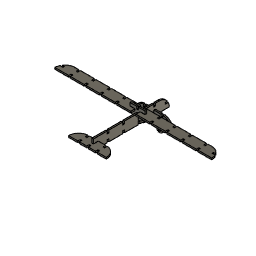
Pressfit Construction Kit v5 (Autodesk Fusion 360 design; units mm, degrees)
Autodesk Fusion 360 part; units mm, degrees
sketch "Sketch1" plane through (0, 0, 0) normal (0, 0, 1) x (1, 0, 0)
  line L0 (75, -10) -> (-75, -10)
  line L1 (-55, 10) -> (75, 10)
  arc A0 (-55, 10) -> (-75, -10) centre (-55, -10) ccw
  line L2 (0, 48.6759) -> (0, -48.6759)
  arc A1 (75, -10) -> (55, 10) centre (55, -10) ccw
  line L3 (-47.4, -10) -> (-44.4, -10)
  line L4 (-44.4, -10) -> (-44.4, -5)
  line L5 (-44.4, -5) -> (-47.4, -5)
  line L6 (-47.4, -5) -> (-47.4, -10)
  line L7 (-13.8, -5) -> (-16.8, -5)
  line L8 (-16.8, -10) -> (-13.8, -10)
  line L9 (-16.8, -5) -> (-16.8, -10)
  line L10 (-13.8, -10) -> (-13.8, -5)
  line L11 (16.8, -5) -> (13.8, -5)
  line L12 (13.8, -10) -> (16.8, -10)
  line L13 (13.8, -5) -> (13.8, -10)
  line L14 (16.8, -10) -> (16.8, -5)
  line L15 (47.4, -5) -> (44.4, -5)
  line L16 (44.4, -10) -> (47.4, -10)
  line L17 (44.4, -5) -> (44.4, -10)
  line L18 (47.4, -10) -> (47.4, -5)
  line L19 (-75, -10) -> (-75, 10) construction
  line L20 (-47.4, -7.5) -> (-75, -7.5) construction
  line L21 (47.4, -7.5) -> (75, -7.5) construction
  line L22 (75, -10) -> (75, 10)
  line L23 (-44.4, -7.5) -> (-16.8, -7.5) construction
  line L24 (-13.8, -7.5) -> (13.8, -7.5) construction
  line L25 (16.8, -7.5) -> (44.4, -7.5) construction
  line L26 (-89.7829, 0) -> (89.7829, 0)
  line L27 (16.8, 5) -> (13.8, 5)
  line L28 (13.8, 10) -> (16.8, 10)
  line L29 (-16.8, 5) -> (-16.8, 10)
  line L30 (-44.4, 10) -> (-44.4, 5)
  line L31 (-13.8, 5) -> (-16.8, 5)
  line L32 (44.4, 5) -> (44.4, 10)
  line L33 (-16.8, 10) -> (-13.8, 10)
  line L34 (16.8, 10) -> (16.8, 5)
  line L35 (13.8, 5) -> (13.8, 10)
  line L36 (-44.4, 5) -> (-47.4, 5)
  line L37 (47.4, 5) -> (44.4, 5)
  line L38 (-47.4, 5) -> (-47.4, 10)
  line L39 (44.4, 10) -> (47.4, 10)
  line L40 (-47.4, 10) -> (-44.4, 10)
  line L41 (-13.8, 10) -> (-13.8, 5)
  line L42 (47.4, 10) -> (47.4, 5)
  line L43 (-67.3205, -1.5) -> (-77.3205, -1.5)
  line L44 (-77.3205, -1.5) -> (-77.3205, 1.5)
  line L45 (-77.3205, 1.5) -> (-67.3205, 1.5)
  line L46 (-67.3205, 1.5) -> (-67.3205, -1.5)
  line L47 (-67.3205, -1.5) -> (-77.3205, 1.5) construction
  line L48 (-77.3205, -1.5) -> (-67.3205, 1.5) construction
  line L49 (75, 1.5) -> (70, 1.5)
  line L50 (70, 1.5) -> (70, -1.5)
  line L51 (70, -1.5) -> (75, -1.5)
  line L52 (75, -1.5) -> (75, 1.5)
  point P0 (44.4, 7.5)
  point P1 (-13.8, 7.5)
  point P2 (13.8, 7.5)
  point P3 (47.4, 7.5)
  point P4 (-16.8, 7.5)
  point P5 (-44.4, 7.5)
  point P6 (-47.4, 7.5)
  point P7 (16.8, 7.5)
  point P8 (55, 10)
  point P9 (-55, 10)
  point P10 (-72.3205, 0)
  dimension "d3" = 150
  dimension "d4" = 20
  dimension "d5" = 20
  dimension "d6" = 10
  dimension "d7" = 110
  dimension "d12" = 3
  dimension "d13" = 5
  dimension "d27" = 3
  dimension "d28" = 10
  dimension "d29" = 5
  dimension "d30" = 3
  constraint horizontal L0
  constraint parallel L0 L1
  constraint perpendicular L0 L2
  constraint midpoint origin L2
  constraint symmetric L0.end L2 L0.start
  constraint symmetric L1.start L2 P8
  constraint symmetric A0 L2 A1
  constraint coincident L0 A0.centre
  constraint horizontal L3
  constraint vertical L4
  constraint horizontal L5
  constraint vertical L6
  constraint coincident L0 L3.start
  constraint equal L5 L7
  constraint equal L7 L11
  constraint equal L11 L15
  constraint collinear L5 L7
  constraint collinear L7 L11
  constraint collinear L11 L15
  constraint parallel L4 L9
  constraint parallel L4 L10
  constraint parallel L10 L14
  constraint parallel L6 L13
  constraint parallel L14 L17
  constraint parallel L9 L18
  constraint tangent A0 L19
  constraint midpoint L6 L20.start
  constraint coincident L19 L20.end
  constraint perpendicular L19 L20
  constraint symmetric L2 L19.end L1.end
  constraint symmetric L2 L20.end L21.end
  constraint horizontal L21
  constraint coincident L18 L21.start
  constraint midpoint L4 L23.start
  constraint midpoint L9 L23.end
  constraint perpendicular L9 L23
  constraint midpoint L10 L24.start
  constraint midpoint L13 L24.end
  constraint perpendicular L13 L24
  constraint midpoint L14 L25.start
  constraint midpoint L17 L25.end
  constraint perpendicular L17 L25
  constraint equal L23 L24
  constraint equal L24 L25
  constraint equal L20 L21
  constraint equal L21 L25
  constraint midpoint origin L26
  constraint horizontal L26
  constraint symmetric A0.centre L26 P9
  constraint symmetric A1.centre L26 A1.end
  constraint symmetric L3.start L26 L38.end
  constraint symmetric L3.end L26 L30.start
  constraint symmetric L4.end L26 L30.end
  constraint symmetric L5.end L26 L36.end
  constraint symmetric L7.start L26 L31.start
  constraint symmetric L7.end L26 L29.start
  constraint symmetric L8.end L26 L33.end
  constraint symmetric L8.start L26 L29.end
  constraint symmetric L11.start L26 L27.start
  constraint symmetric L11.end L26 L27.end
  constraint symmetric L12.end L26 L28.end
  constraint symmetric L12.start L26 L28.start
  constraint symmetric L15.start L26 L37.start
  constraint symmetric L15.end L26 L32.start
  constraint symmetric L16.end L26 L39.end
  constraint symmetric L16.start L26 L32.end
  constraint symmetric L20.start L26 P6
  constraint symmetric L21.start L26 P3
  constraint symmetric L23.start L26 P5
  constraint symmetric L23.end L26 P4
  constraint symmetric L25.end L26 P0
  constraint collinear L0 L12
  constraint collinear L0 L16
  constraint horizontal L43
  constraint perpendicular L43 L44
  constraint parallel L43 L45
  constraint parallel L44 L46
  constraint coincident L47 P10
  constraint coincident L48 P10
  constraint coincident A0 P10
  constraint coincident L26 P10
  constraint coincident L1 P8
  constraint horizontal L49
  constraint vertical L50
  constraint horizontal L51
  constraint vertical L52
  constraint coincident L22 L49.start
  constraint midpoint L22 L52
  measures "d3" distance of L0.start L0.end
  measures "d4" distance of L0 L1
  measures "d5" radius of A0
  measures "d6" distance of L0 origin
  measures "d12" distance of L3.start L3.end
  measures "d13" distance of L3.start L5.end
  measures "d27" distance of L43.end L44.end
  measures "d28" distance of L44.end L45.end
  measures "d29" distance of L49.start L49.end
  measures "d30" distance of L49.end L50.end
extrude "Extrude1" add sketch "Sketch1" along normal mid plane 3 contours L0 L2 A1 L11 L13 L14 L15 L17 L18 L26 L50 L51 | A1 L22 L51 | L1 L2 A1 L26 L27 L32 L34 L35 L37 L42 L49 L50 | L1 A1 L22 L49 | L1 A0 L2 L26 L29 L30 L31 L36 L38 L41 L45 L46 | L0 A0 L2 L4 L5 L6 L7 L9 L10 L26 L43 L46 makes body 1
sketch "Sketch6" plane through (0, 0, 1.5) normal (0, 0, 1) x (-1, 0, 0)
  line L0 (-75, -1.5) -> (-75, -10)
  line L1 (-75, -10) -> (-47.4, -10)
  line L2 (-47.4, -10) -> (-47.4, -5)
  line L3 (-47.4, -5) -> (-44.4, -5)
  line L4 (-44.4, -5) -> (-44.4, -10)
  line L5 (-44.4, -10) -> (-16.8, -10)
  line L6 (-16.8, -10) -> (-16.8, -5)
  line L7 (-16.8, -5) -> (-13.8, -5)
  line L8 (-13.8, -5) -> (-13.8, -10)
  line L9 (-13.8, -10) -> (13.8, -10)
  line L10 (13.8, -10) -> (13.8, -5)
  line L11 (13.8, -5) -> (16.8, -5)
  line L12 (16.8, -5) -> (16.8, -10)
  line L13 (16.8, -10) -> (44.4, -10)
  line L14 (44.4, -10) -> (44.4, -5)
  line L15 (44.4, -5) -> (47.4, -5)
  line L16 (47.4, -5) -> (47.4, -10)
  line L17 (47.4, -10) -> (55, -10)
  arc A0 (55, -10) -> (71.3631, -1.5) centre (55, 10) ccw
  line L18 (71.3631, -1.5) -> (67.3205, -1.5)
  line L19 (67.3205, -1.5) -> (67.3205, 1.5)
  line L20 (67.3205, 1.5) -> (73.1039, 1.5)
  arc A1 (73.1039, 1.5) -> (75, 10) centre (55, 10) ccw
  line L21 (75, 10) -> (47.4, 10)
  line L22 (47.4, 10) -> (47.4, 5)
  line L23 (47.4, 5) -> (44.4, 5)
  line L24 (44.4, 5) -> (44.4, 10)
  line L25 (44.4, 10) -> (16.8, 10)
  line L26 (16.8, 10) -> (16.8, 5)
  line L27 (16.8, 5) -> (13.8, 5)
  line L28 (13.8, 5) -> (13.8, 10)
  line L29 (13.8, 10) -> (-13.8, 10)
  line L30 (-13.8, 10) -> (-13.8, 5)
  line L31 (-13.8, 5) -> (-16.8, 5)
  line L32 (-16.8, 5) -> (-16.8, 10)
  line L33 (-16.8, 10) -> (-44.4, 10)
  line L34 (-44.4, 10) -> (-44.4, 5)
  line L35 (-44.4, 5) -> (-47.4, 5)
  line L36 (-47.4, 5) -> (-47.4, 10)
  line L37 (-47.4, 10) -> (-75, 10)
  line L38 (-75, 10) -> (-75, 1.5)
  line L39 (-75, 1.5) -> (-70, 1.5)
  line L40 (-70, 1.5) -> (-70, -1.5)
  line L41 (-70, -1.5) -> (-75, -1.5)
sketch "Sketch3" plane through (0, 0, 0) normal (0, 0, 1) x (1, 0, 0)
  circle A0 centre (0, 0) radius 15
  line L0 (0, 13.5) -> (0, -13.5) construction
  line L1 (1.5, 10) -> (-1.5, 10)
  line L2 (-1.5, 10) -> (-1.5, 20)
  line L3 (-1.5, 20) -> (1.5, 20)
  line L4 (1.5, 20) -> (1.5, 10)
  line L5 (1.5, 10) -> (-1.5, 20) construction
  line L6 (-1.5, 10) -> (1.5, 20) construction
  line L7 (-1.5, -20) -> (-1.5, -10)
  line L8 (1.5, -10) -> (1.5, -20)
  line L9 (-1.5, -10) -> (1.5, -20) construction
  line L10 (1.5, -10) -> (-1.5, -20) construction
  line L11 (1.5, -20) -> (-1.5, -20)
  line L12 (-1.5, -10) -> (1.5, -10)
  line L13 (-7.5, -1.5) -> (-22.5, -1.5)
  line L14 (-22.5, -1.5) -> (-22.5, 1.5)
  line L15 (-22.5, 1.5) -> (-7.5, 1.5)
  line L16 (-7.5, 1.5) -> (-7.5, -1.5)
  line L17 (-7.5, -1.5) -> (-22.5, 1.5) construction
  line L18 (-22.5, -1.5) -> (-7.5, 1.5) construction
  line L19 (-37, 0) -> (37, 0) construction
  line L20 (0, 15) -> (7.5, 15)
  line L21 (7.5, 15) -> (7.5, -15)
  line L22 (7.5, -15) -> (0, -15)
  line L23 (7.5, 1.5) -> (7.5, -1.5)
  line L24 (12.5, -1.5) -> (2.5, -1.5)
  line L25 (2.5, -1.5) -> (2.5, 1.5)
  line L26 (2.5, 1.5) -> (12.5, 1.5)
  line L27 (12.5, 1.5) -> (12.5, -1.5)
  line L28 (12.5, -1.5) -> (2.5, 1.5) construction
  line L29 (2.5, -1.5) -> (12.5, 1.5) construction
  point P0 (0, 15)
  point P1 (0, -15)
  point P2 (0, -13.5)
  point P3 (75, 10)
  point P4 (75, -10)
  point P5 (-15, 0)
  point P6 (7.5, 0)
  dimension "d20" = 30
  dimension "d21" = 3
  dimension "d22" = 10
  dimension "d24" = 360
  dimension "d47" = 20
  dimension "d64" = 3
  dimension "d65" = 15
  dimension "d116" = 3
  dimension "d117" = 10
  constraint coincident A0.centre origin
  constraint vertical L0
  constraint midpoint A0.centre L0
  constraint horizontal L1
  constraint perpendicular L1 L2
  constraint parallel L1 L3
  constraint parallel L2 L4
  constraint coincident L5 P0
  constraint coincident L6 P0
  constraint coincident L0 P0
  constraint coincident A0 P0
  constraint horizontal L13
  constraint perpendicular L13 L14
  constraint parallel L13 L15
  constraint parallel L14 L16
  constraint coincident L17 P5
  constraint coincident L18 P5
  constraint coincident A0 P5
  constraint horizontal L19
  constraint midpoint A0.centre L19
  constraint coincident P5 L19
  constraint coincident P0 L20.start
  constraint tangent A0 L20
  constraint coincident P1 L22.end
  constraint tangent A0 L22
  constraint parallel L20 L22
  constraint perpendicular L20 L21
  constraint symmetric L0 L13.start L23.end
  constraint symmetric L0 L15.end L23.start
  constraint collinear L21 L23
  constraint horizontal L24
  constraint perpendicular L24 L25
  constraint parallel L24 L26
  constraint parallel L25 L27
  constraint coincident L28 P6
  constraint coincident L29 P6
  constraint midpoint L23 P6
  measures "d20" diameter of A0
  measures "d21" distance of L2.end L3.end
  measures "d22" distance of L1.end L2.end
  measures "d47" distance of P3 P4
  measures "d64" distance of L13.end L14.end
  measures "d65" distance of L13.start L13.end
  measures "d116" distance of L24.end L25.end
  measures "d117" distance of L25.end L26.end
extrude "Extrude2" add sketch "Sketch3" along normal mid plane 3 separate body contours A0 L1 L2 L4 L7 L8 L12 L13 L15 L16 L21 L24 L25 L26 | A0 L4 L20 L21 | A0 L8 L21 L22 makes body 2
sketch "Sketch7" plane through (0, 0, 1.5) normal (0, 0, 1) x (-1, 0, 0)
  line L0 (-7.5, 1.5) -> (-2.5, 1.5)
  line L1 (-2.5, 1.5) -> (-2.5, -1.5)
  line L2 (-2.5, -1.5) -> (-7.5, -1.5)
  line L3 (-7.5, -1.5) -> (-7.5, -15)
  line L4 (-7.5, -15) -> (-1.5, -15)
  line L5 (-1.5, -15) -> (-1.5, -10)
  line L6 (-1.5, -10) -> (1.5, -10)
  line L7 (1.5, -10) -> (1.5, -14.9248)
  arc A0 (1.5, -14.9248) -> (14.9248, -1.5) centre (0, 0) ccw
  line L8 (14.9248, -1.5) -> (7.5, -1.5)
  line L9 (7.5, -1.5) -> (7.5, 1.5)
  line L10 (7.5, 1.5) -> (14.9248, 1.5)
  arc A1 (14.9248, 1.5) -> (1.5, 14.9248) centre (0, 0) ccw
  line L11 (1.5, 14.9248) -> (1.5, 10)
  line L12 (1.5, 10) -> (-1.5, 10)
  line L13 (-1.5, 10) -> (-1.5, 15)
  line L14 (-1.5, 15) -> (-7.5, 15)
  line L15 (-7.5, 15) -> (-7.5, 1.5)
copy_body "Body->Comp1" bodies 1 removing the originals makes body 3 in component "fintype"
sketch "Sketch4" plane through (0, 0, 0) normal (0, 0, 1) x (1, 0, 0)
  line L0 (37.5, -10) -> (-37.5, -10)
  line L1 (-17.5, 10) -> (17.0754, 10)
  arc A0 (-17.5, 10) -> (-37.5, -10) centre (-17.5, -10) ccw
  arc A1 (-0.1556, -0.0415) -> (-0.2123, 0.0566) centre (-17.5, -10) ccw
  line L2 (-0.2123, 35.0566) -> (-0.2123, -34.9434) construction
  line L3 (-45.2123, 0.0566) -> (44.7877, 0.0566) construction
  arc A2 (37.0754, -10) -> (17.0754, 10) centre (17.0754, -10) ccw
  line L4 (-19.2661, -10) -> (-16.2661, -10)
  line L5 (-16.2661, -10) -> (-16.2661, -5)
  line L6 (-16.2661, -5) -> (-19.2661, -5)
  line L7 (-19.2661, -5) -> (-19.2661, -10)
  line L8 (1.2873, -10) -> (-1.7127, -10)
  line L9 (-1.7127, -10) -> (-1.7127, -5)
  line L10 (-1.7127, -5) -> (1.2873, -5)
  line L11 (1.2873, -5) -> (1.2873, -10)
  line L12 (18.8407, -10) -> (15.8407, -10)
  line L13 (15.8407, -10) -> (15.8407, -5)
  line L14 (15.8407, -5) -> (18.8407, -5)
  line L15 (18.8407, -5) -> (18.8407, -10)
  line L16 (-37.5, -10) -> (-37.5, 10) construction
  line L17 (37.0754, -10) -> (37.0754, 10) construction
  line L18 (-37.5, -7.3291) -> (-19.2661, -7.5) construction
  line L19 (-16.2661, -7.5) -> (-1.7127, -7.5) construction
  line L20 (1.2873, -7.5) -> (15.8407, -7.5) construction
  line L21 (18.8407, -7.5) -> (37.0754, -7.5) construction
  line L22 (-16.2661, 7.6132) -> (-1.7127, 7.6132) construction
  line L23 (-19.2661, 5.1132) -> (-19.2661, 10.1132)
  line L24 (1.2873, 5.1132) -> (1.2873, 10.1132)
  line L25 (18.8407, 5.1132) -> (18.8407, 10.1132)
  line L26 (-16.2661, 5.1132) -> (-19.2661, 5.1132)
  line L27 (-19.2661, 10.1132) -> (-16.2661, 10.1132)
  line L28 (18.8407, 10.1132) -> (15.8407, 10.1132)
  line L29 (-16.2661, 10.1132) -> (-16.2661, 5.1132)
  line L30 (-1.7127, 10.1132) -> (-1.7127, 5.1132)
  line L31 (1.2873, 10.1132) -> (-1.7127, 10.1132)
  line L32 (15.8407, 10.1132) -> (15.8407, 5.1132)
  line L33 (1.2873, 7.6132) -> (15.8407, 7.6132) construction
  line L34 (-1.7127, 5.1132) -> (1.2873, 5.1132)
  line L35 (15.8407, 5.1132) -> (18.8407, 5.1132)
  point P0 (18.8407, 7.6132)
  point P1 (-19.2661, 7.6132)
  point P2 (17.0754, 10.1132)
  point P3 (-17.5, 10.1132)
  point P4 (-17.5, 10.1132)
  dimension "d72" = 75
  dimension "d73" = 20
  dimension "d74" = 20
  dimension "d75" = 10.0566
  dimension "d76" = 17.2877
  dimension "d77" = 3
  dimension "d78" = 5
  constraint horizontal L0
  constraint parallel L0 L1
  constraint tangent L1 A0
  constraint concentric A0 A1
  constraint perpendicular L0 L2
  constraint midpoint L2 L3
  constraint midpoint A1.end L3
  constraint symmetric L0.end L2 A2.start
  constraint symmetric L1.start L2 L1.end
  constraint symmetric A0 L2 A2
  constraint horizontal L4
  constraint vertical L5
  constraint horizontal L6
  constraint vertical L7
  constraint coincident L0 L4.start
  constraint horizontal L8
  constraint vertical L9
  constraint horizontal L10
  constraint vertical L11
  constraint coincident L0 L8.start
  constraint horizontal L12
  constraint vertical L13
  constraint horizontal L14
  constraint vertical L15
  constraint coincident L0 L12.start
  constraint collinear L6 L10
  constraint collinear L10 L14
  constraint tangent A0 L16
  constraint symmetric L2 L16.end L17.end
  constraint coincident L16 L18.start
  constraint midpoint L7 L18.end
  constraint midpoint L5 L19.start
  constraint midpoint L9 L19.end
  constraint midpoint L11 L20.start
  constraint midpoint L13 L20.end
  constraint midpoint L15 L21.start
  constraint coincident L17 L21.end
  constraint perpendicular L17 L21
  constraint equal L19 L20
  constraint equal L6 L10
  constraint equal L10 L14
  constraint equal L18 L21
  constraint symmetric A0.centre L3 P3
  constraint symmetric A0.centre L3 P4
  constraint symmetric L3 A2.centre P2
  constraint symmetric L3 L4.start L23.end
  constraint symmetric L3 L4.end L27.end
  constraint symmetric L3 L5.end L26.start
  constraint symmetric L3 L6.end L23.start
  constraint symmetric L3 L8.start L24.end
  constraint symmetric L3 L8.end L30.start
  constraint symmetric L3 L9.end L30.end
  constraint symmetric L3 L10.end L24.start
  constraint symmetric L3 L12.start L25.end
  constraint symmetric L3 L12.end L28.end
  constraint symmetric L3 L13.end L32.end
  constraint symmetric L3 L14.end L25.start
  constraint symmetric L3 L18.end P1
  constraint symmetric L3 L19.start L22.start
  constraint symmetric L3 L19.end L22.end
  constraint symmetric L3 L20.start L33.start
  constraint symmetric L3 L20.end L33.end
  constraint symmetric L3 L21.start P0
  measures "d72" distance of L0.start L0.end
  measures "d73" distance of L0 L1
  measures "d74" radius of A0
  measures "d75" distance of L0 L3
  measures "d76" distance of A0.centre L2
  measures "d77" distance of L5.end L6.end
  measures "d78" distance of L4.start L6.end
extrude "Extrude3" add sketch "Sketch4" along normal mid plane 3 separate body contours L0 L1 A0 A2 L5 L6 L7 L9 L10 L11 L13 L14 L15 L23 L24 L25 L26 L29 L30 L32 L34 L35 makes body 4
sketch "Sketch8" plane through (0, 0, 1.5) normal (0, 0, 1) x (-1, 0, 0)
  line L0 (16.2661, -10) -> (16.2661, -5.1132)
  line L1 (16.2661, -5.1132) -> (19.2661, -5.1132)
  line L2 (19.2661, -5.1132) -> (19.2661, -9.9219)
  arc A0 (19.2661, -9.9219) -> (37.5, 10) centre (17.5, 10) ccw
  line L3 (37.5, 10) -> (19.2661, 10)
  line L4 (19.2661, 10) -> (19.2661, 5)
  line L5 (19.2661, 5) -> (16.2661, 5)
  line L6 (16.2661, 5) -> (16.2661, 10)
  line L7 (16.2661, 10) -> (1.7127, 10)
  line L8 (1.7127, 10) -> (1.7127, 5)
  line L9 (1.7127, 5) -> (-1.2873, 5)
  line L10 (-1.2873, 5) -> (-1.2873, 10)
  line L11 (-1.2873, 10) -> (-15.8407, 10)
  line L12 (-15.8407, 10) -> (-15.8407, 5)
  line L13 (-15.8407, 5) -> (-18.8407, 5)
  line L14 (-18.8407, 5) -> (-18.8407, 10)
  line L15 (-18.8407, 10) -> (-37.0754, 10)
  arc A1 (-37.0754, 10) -> (-18.8407, -9.9219) centre (-17.0754, 10) ccw
  line L16 (-18.8407, -9.9219) -> (-18.8407, -5.1132)
  line L17 (-18.8407, -5.1132) -> (-15.8407, -5.1132)
  line L18 (-15.8407, -5.1132) -> (-15.8407, -10)
  line L19 (-15.8407, -10) -> (-1.2873, -10)
  line L20 (-1.2873, -10) -> (-1.2873, -5.1132)
  line L21 (-1.2873, -5.1132) -> (1.7127, -5.1132)
  line L22 (1.7127, -5.1132) -> (1.7127, -10)
  line L23 (1.7127, -10) -> (16.2661, -10)
copy_body "Body->Comp3" bodies 4 removing the originals makes body 5 in component "FIN_2"
copy_body "Body->Comp4" bodies 2 removing the originals makes body 6 in component "CONNECTOR"
sketch "Sketch5" plane through (0, 0, 0) normal (0, 0, 1) x (1, 0, 0)
  circle A0 centre (0, 0) radius 10
  line L0 (0, 18.5305) -> (0, -18.5305)
  line L1 (-16.5, 0) -> (16.5, 0)
  line L2 (1.5, 5) -> (-1.5, 5)
  line L3 (-1.5, 5) -> (-1.5, 15)
  line L4 (-1.5, 15) -> (1.5, 15)
  line L5 (1.5, 15) -> (1.5, 5)
  line L6 (1.5, 5) -> (-1.5, 15) construction
  line L7 (-1.5, 5) -> (1.5, 15) construction
  line L8 (-3.5801, -3.799) -> (-12.2404, -8.799)
  line L9 (-12.2404, -8.799) -> (-13.7404, -6.201)
  line L10 (-13.7404, -6.201) -> (-5.0801, -1.201)
  line L11 (-3.5801, -3.799) -> (-13.7404, -6.201) construction
  line L12 (-5.0801, -1.201) -> (-3.5801, -3.799)
  line L13 (-5.0801, -1.201) -> (-12.2404, -8.799) construction
  line L14 (5.0801, -1.201) -> (13.7404, -6.201)
  line L15 (13.7404, -6.201) -> (12.2404, -8.799)
  line L16 (12.2404, -8.799) -> (3.5801, -3.799)
  line L17 (5.0801, -1.201) -> (12.2404, -8.799) construction
  line L18 (3.5801, -3.799) -> (5.0801, -1.201)
  line L19 (3.5801, -3.799) -> (13.7404, -6.201) construction
  point P0 (0, 10)
  point P1 (-16.0479, -9.2652)
  point P2 (-8.6603, -5)
  point P3 (16.0479, -9.2652)
  point P4 (8.6603, -5)
  dimension "d101" = 20
  dimension "d102" = 3
  dimension "d103" = 10
  dimension "d105" = 360
  constraint coincident A0.centre origin
  constraint vertical L0
  constraint perpendicular L0 L1
  constraint midpoint A0.centre L1
  constraint midpoint A0.centre L0
  constraint horizontal L2
  constraint perpendicular L2 L3
  constraint parallel L2 L4
  constraint parallel L3 L5
  constraint coincident L6 P0
  constraint coincident L7 P0
  constraint coincident A0 P0
  constraint coincident L0 P0
  measures "d101" diameter of A0
  measures "d102" distance of L3.end L4.end
  measures "d103" distance of L2.end L3.end
extrude "Extrude4" add sketch "Sketch5" along normal mid plane 3 separate body contours A0 L0 L1 L2 L5 | A0 L0 L1 L14 L16 L18 | A0 L0 L1 L2 L3 | A0 L0 L1 L8 L10 L12 makes body 7
sketch "Sketch9" plane through (0, 0, -1.5) normal (0, 0, -1) x (1, 0, 0)
  line L0 (5.0801, 1.201) -> (3.5801, 3.799)
  line L1 (3.5801, 3.799) -> (7.8123, 6.2425)
  arc A0 (7.8123, 6.2425) -> (-7.8123, 6.2425) centre (0, 0) ccw
  line L2 (-7.8123, 6.2425) -> (-3.5801, 3.799)
  line L3 (-3.5801, 3.799) -> (-5.0801, 1.201)
  line L4 (-5.0801, 1.201) -> (-9.3123, 3.6444)
  arc A1 (-9.3123, 3.6444) -> (-1.5, -9.8869) centre (0, 0) ccw
  line L5 (-1.5, -9.8869) -> (-1.5, -5)
  line L6 (-1.5, -5) -> (1.5, -5)
  line L7 (1.5, -5) -> (1.5, -9.8869)
  arc A2 (1.5, -9.8869) -> (9.3123, 3.6444) centre (0, 0) ccw
  line L8 (9.3123, 3.6444) -> (5.0801, 1.201)
copy_body "Body->Comp5" bodies 7 removing the originals makes body 8 in component "WHEEL"
component "fintype" placed x (1, 0, 0) y (0, 1, 0) z (0, 0, 1) at (-17.6868, -6.8741, 6.7291)
component "fintype" placed x (0, -1, 0) y (0, 0, 1) z (-1, 0, 0) at (62.3132, -22.1741, -5.7709)
component "fintype" placed x (-1, 0, 0) y (0, 1, 0) z (0, 0, -1) at (142.3132, -6.8741, 6.7291)
component "FIN_2" placed x (1, 0, 0) y (0, 1, 0) z (0, 0, 1) at (62.5259, -97.2873, -5.7709)
component "CONNECTOR" placed x (0, 0, 1) y (1, 0, 0) z (0, 1, 0) at (62.3132, -6.8741, 6.7291)
component "FIN_2" placed x (1, 0, 0) y (0, 0, 1) z (0, -1, 0) at (62.5259, 23.7259, -15.8842)
component "WHEEL" placed x (0, 0.5, 0.866025) y (0, 0.866025, -0.5) z (-1, 0, 0) at (44.7598, 23.7259, -25.8842)
component "WHEEL" placed x (0, 0.5, 0.866025) y (0, 0.866025, -0.5) z (-1, 0, 0) at (79.8666, 23.7259, -25.8842)
equation "kerf = 0.25 mm"
equation "thickness = 3 mm"
equation "d12 = thickness"
equation "d13 = d4 * ( 1 / 4 )"
equation "d18 = thickness"
equation "d21 = thickness"
equation "d22 = ( d47 * ( 1 / 4 ) * 2 )"
equation "d25 = thickness"
equation "d27 = thickness"
equation "d28 = ( d4 * ( 1 / 4 ) ) * 2"
equation "d29 = d13"
equation "d30 = thickness"
equation "d64 = thickness"
equation "d65 = ( d20 * ( 1 / 4 ) ) * 2"
equation "d77 = thickness"
equation "d78 = d73 * ( 1 / 4 )"
equation "d79 = thickness"
equation "d102 = thickness"
equation "d103 = ( d101 * ( 1 / 4 ) ) * 2"
equation "d106 = thickness"
equation "d116 = thickness"
equation "d117 = d22"
named bodies: "WHEEL"
